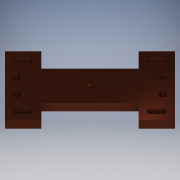
# Autodesk Inventor part: mount-base
Saved by Autodesk Inventor 2017 SP1 (Build 210196100, 196)
## iProperties
Created: 2017-02-03
Part Number: mount-base
Material: Copper
Document SubType Name: Modeling
Designer: Alex
Density: 8.94 g/cm^3
Appearance: Copper - Polished
Author: Alex
Autodesk Inventor part; units mm, degrees
ref_plane "YZ Plane" through (0, 0, 0) normal (1, 0, 0) x (0, 1, 0)
ref_plane "XZ Plane" through (0, 0, 0) normal (0, 1, 0) x (-1, 0, 0)
ref_plane "XY Plane" through (0, 0, 0) normal (0, 0, 1) x (1, 0, 0)
sketch "Sketch1" plane through (0, 0, 0) normal (0, 1, 0) x (-1, 0, 0)
  line L0 (-10, 20) -> (-10, 0)
  line L1 (10, 0) -> (10, 20)
  line L2 (20, 20) -> (10, 20)
  line L3 (-10, 20) -> (-20, 20)
  line L4 (20, 20) -> (20, 35)
  line L5 (-20, 35) -> (-20, 20)
  line L6 (20, 35) -> (-20, 35)
  line L7 (10, 0) -> (-10, 0) construction
  line L8 (10, 20) -> (-10, 20) construction
  line L9 (0, 20) -> (0, 0) construction
  line L10 (10, 15) -> (-10, 15) construction
  line L11 (10, 15) -> (0, 15) construction
  line L12 (0, 15) -> (-10, 15) construction
  line L13 (15, 35) -> (15, 27.5) construction
  line L14 (15, 27.5) -> (15, 20) construction
  line L15 (-15, 35) -> (-15, 27.5) construction
  line L16 (-15, 27.5) -> (-15, 20) construction
  line L17 (0, 15) -> (5, 15) construction
  line L18 (0, 15) -> (-5, 15) construction
  line L19 (5.1791, 30) -> (-4.8209, 30)
  line L20 (20, 27.5) -> (15, 27.5)
  line L21 (-20, 27.5) -> (-15, 27.5)
  line L22 (-10, -20) -> (-10, 0)
  line L23 (10, 0) -> (10, -20)
  line L24 (20, -20) -> (10, -20)
  line L25 (-10, -20) -> (-20, -20)
  line L26 (20, -20) -> (20, -35)
  line L27 (-20, -35) -> (-20, -20)
  line L28 (20, -35) -> (-20, -35)
  line L29 (10, -20) -> (-10, -20) construction
  line L30 (0, -20) -> (0, 0) construction
  line L31 (10, -15) -> (-10, -15) construction
  line L32 (10, -15) -> (0, -15) construction
  line L33 (0, -15) -> (-10, -15) construction
  line L34 (15, -35) -> (15, -27.5) construction
  line L35 (15, -27.5) -> (15, -20) construction
  line L36 (-15, -35) -> (-15, -27.5) construction
  line L37 (-15, -27.5) -> (-15, -20) construction
  line L38 (0, -15) -> (5, -15) construction
  line L39 (0, -15) -> (-5, -15) construction
  line L40 (5.1791, -30) -> (-4.8209, -30)
  line L41 (20, -27.5) -> (15, -27.5)
  line L42 (-20, -27.5) -> (-15, -27.5)
  dimension "outerW" = 15
  dimension "d84" = 5
  dimension "d127" = 20
  dimension "d128" = 35
  dimension "d129" = 5
  constraints: 86 end point, 22 symmetric about line, 8 midpoint, 8 point on line, 4 collinear, 2 horizontal, 2 parallel, 2 perpendicular, 1 vertical
  measures "outerW" distance between parallel lines of L6 L3
  measures "d84" distance between parallel lines of L10 L8
  measures "d127" distance between parallel lines of L0 L1
  measures "d128" distance between parallel lines of L6 L7
  measures "d129" distance between parallel lines of L6 L19
extrude "Extrusion1" add sketch "Sketch1" along normal blind 5
sketch "Sketch8" plane through (0, 5, 0) normal (0, 1, 0) x (1, 0, 0)
  line L0 (-10, -20) -> (-10, 20) projected
  line L1 (-10, 20) -> (-20, 20) projected
  line L2 (-20, 20) -> (-20, 35) projected
  line L3 (-20, 35) -> (20, 35) projected
  line L4 (20, 35) -> (20, 20) projected
  line L5 (20, 20) -> (10, 20) projected
  line L6 (10, 20) -> (10, -20) projected
  line L7 (10, -20) -> (20, -20) projected
  line L8 (20, -20) -> (20, -35) projected
  line L9 (20, -35) -> (-20, -35) projected
  line L10 (-20, -35) -> (-20, -20) projected
  line L11 (-20, -20) -> (-10, -20) projected
  line L12 (-20, -20) -> (-20, -35) projected
  line L13 (-20, -27.5) -> (-15, -27.5)
  line L14 (20, -35) -> (20, -20) projected
  line L15 (20, -27.5) -> (15, -27.5)
  line L16 (20, -30) -> (-20, -30)
  line L17 (-5, -30) -> (5, -30)
  line L18 (5, -30) -> (5, -35)
  line L19 (-5, -35) -> (-5, -30)
  line L20 (-5, -30) -> (0, -30)
  line L21 (-10, 20) -> (-10, -20) projected
  line L22 (-10, 0) -> (10, 0)
  line L23 (10, 20) -> (20, 20)
  line L24 (20, 20) -> (20, 35)
  line L25 (20, 35) -> (-20, 35)
  line L26 (-20, 35) -> (-20, 20)
  line L27 (-20, 20) -> (-10, 20)
  line L28 (-20, 20) -> (-20, 35)
  line L29 (-20, 27.5) -> (-15, 27.5)
  line L30 (20, 35) -> (20, 20)
  line L31 (20, 27.5) -> (15, 27.5)
  line L32 (20, 30) -> (-20, 30)
  line L33 (-5, 30) -> (5, 30)
  line L34 (5, 30) -> (5, 35)
  line L35 (-5, 35) -> (-5, 30)
  line L36 (-5, 30) -> (0, 30)
  point P0 (0, 0)
  point P1 (0, -35)
  point P2 (0, 35)
  dimension "d130" = 5
  constraints: 44 end point, 12 symmetric about line, 8 point on line, 6 midpoint, 3 horizontal, 2 perpendicular, 1 parallel
  measures "d130" distance between parallel lines of L9 L16
hole "Hole12" at (-5, 5, 30) at (-5, 5, -30) at (5, 5, 30) at (5, 5, -30) direction (0, -1, 0) diameter 3.4 end through all clearance for "Socket Head Cap Screw ISO 4762" size "M3" standard "ISO"
sketch "Sketch9" plane through (0, 5, 0) normal (0, 1, 0) x (1, 0, 0)
  circle A0 centre (5, -30) radius 1.7 projected
  circle A1 centre (-5, -30) radius 1.7 projected
  circle A2 centre (-5, 30) radius 1.7 projected
  circle A3 centre (5, 30) radius 1.7 projected
  line L0 (-10, -20) -> (-10, 20) projected
  line L1 (-10, 20) -> (-20, 20) projected
  line L2 (-20, 20) -> (-20, 35) projected
  line L3 (-20, 35) -> (20, 35) projected
  line L4 (20, 35) -> (20, 20) projected
  line L5 (20, 20) -> (10, 20) projected
  line L6 (10, 20) -> (10, -20) projected
  line L7 (10, -20) -> (20, -20) projected
  line L8 (20, -20) -> (20, -35) projected
  line L9 (20, -35) -> (-20, -35) projected
  line L10 (-20, -35) -> (-20, -20) projected
  line L11 (-20, -20) -> (-10, -20) projected
  line L12 (-20, -20) -> (-20, -35) projected
  line L13 (20, -35) -> (20, -20) projected
  line L14 (-20, -35) -> (20, -35) projected
  line L15 (-13.5, -31.5) -> (-16.5, -31.5)
  line L16 (-16.5, -31.5) -> (-16.5, -23.5)
  line L17 (-16.5, -23.5) -> (-13.5, -23.5)
  line L18 (-13.5, -23.5) -> (-13.5, -31.5)
  line L19 (-13.5, -31.5) -> (-16.5, -23.5) construction
  line L20 (-16.5, -31.5) -> (-13.5, -23.5) construction
  line L21 (16.5, -31.5) -> (13.5, -31.5)
  line L22 (13.5, -31.5) -> (13.5, -23.5)
  line L23 (13.5, -23.5) -> (16.5, -23.5)
  line L24 (16.5, -23.5) -> (16.5, -31.5)
  line L25 (16.5, -31.5) -> (13.5, -23.5) construction
  line L26 (13.5, -31.5) -> (16.5, -23.5) construction
  point P0 (0, 0)
  point P1 (-15, -27.5)
  point P2 (15, -27.5)
  dimension "d140" = 3
  dimension "d141" = 8
  dimension "d142" = 3
  dimension "d143" = 8
  constraints: 24 end point, 4 midpoint, 4 parallel, 2 horizontal, 2 perpendicular
  measures "d140" distance of L16.end L17.end
  measures "d141" distance of L15.end L16.end
  measures "d142" distance of L22.end L23.end
  measures "d143" distance of L21.end L22.end
extrude "Extrusion4" cut sketch "Sketch9" against normal through all contours L15 L16 L17 L18 | L21 L22 L23 L24
mirror "Mirror3" about plane through (0, 0, 0) normal (0, 0, 1) of "Extrusion4"
fillet "Fillet4" radius 1.3 16 edges at (-16.5, 2.5, 23.5) (-13.5, 2.5, 23.5) (13.5, 2.5, 23.5) (16.5, 2.5, 23.5) (-16.5, 2.5, 31.5) (-13.5, 2.5, 31.5) (13.5, 2.5, 31.5) (16.5, 2.5, 31.5) (-16.5, 2.5, -31.5) (-13.5, 2.5, -31.5) (-16.5, 2.5, -23.5) (-13.5, 2.5, -23.5) (13.5, 2.5, -23.5) (16.5, 2.5, -23.5) (13.5, 2.5, -31.5) (16.5, 2.5, -31.5)
body "Solid1"
